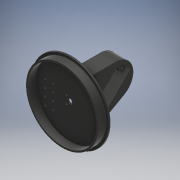
# Autodesk Inventor part: 第一關節
Saved by Autodesk Inventor 2017 (Build 210142000, 142)
## iProperties
Part Number: 第一關節
Material: 熱塑性塑膠樹脂
Document SubType Name: Modeling
Designer: Brian
Density: 1.28 g/cm^3
Appearance: 平滑 - 黑色
Mass: 82.2152 g
Surface Area: 315.278 cm^2
Volume: 64.2306 cm^3
Author: Brian
Autodesk Inventor part; units mm, degrees
ref_plane "YZ Plane" through (0, 0, 0) normal (1, 0, 0) x (0, 1, 0)
ref_plane "XZ Plane" through (0, 0, 0) normal (0, 1, 0) x (-1, 0, 0)
ref_plane "XY Plane" through (0, 0, 0) normal (0, 0, 1) x (1, 0, 0)
sketch "草圖1" plane through (0, 0, 0) normal (0, 1, 0) x (-1, 0, 0)
  circle A0 centre (0, 0) radius 46.75
  circle A1 centre (0, 0) radius 44.75
  dimension "d0" = 93.5
  dimension "d1" = 2
  constraints: 2 centre point, 2 coincident
  measures "d0" diameter of A0
  measures "d1" radial gap between concentric circles of A0 A1
extrude "擠出1" add sketch "草圖1" along normal blind 10
sketch "草圖2" plane through (0, 10, 0) normal (0, 1, 0) x (1, 0, 0)
  circle A0 centre (0, 0) radius 50
  dimension "d4" = 100
  constraints: 1 centre point, 1 coincident
  measures "d4" diameter of A0
extrude "擠出2" add sketch "草圖2" along normal blind 2
sketch "草圖4" plane through (0, 0, 0) normal (1, 0, 0) x (0, 1, 0)
  line L0 (12, -50) -> (12, 50) projected
  line L1 (12, -25.0248) -> (30.0379, -25.0248)
  line L2 (30.0379, -25.0248) -> (30.0379, 11.7448)
  line L3 (30.0379, 11.7448) -> (12, 11.7448)
  line L4 (12, 11.7448) -> (12, -25.0248)
  line L5 (30.0379, -25.0248) -> (72.4644, 17.4017)
  line L6 (72.4644, 17.4017) -> (54.0796, 35.7864)
  line L7 (54.0796, 35.7864) -> (11.6532, -6.64)
  line L8 (11.6532, -6.64) -> (30.0379, -25.0248)
  point P0 (0, 0)
  dimension "d12" = 45
  dimension "d13" = 26
  dimension "d14" = 60
  constraints: 16 end point, 4 parallel, 2 perpendicular, 2 point on line, 1 horizontal
  measures "d12" angle of L2 L7
  measures "d13" distance of L5.end L6.end
  measures "d14" distance of L1.end L5.end
extrude "擠出4" add sketch "草圖4" along normal blind 5
fillet "圓角1" radius 10 1 edges at (2.5, 30.0379, 11.7448)
fillet "圓角2" radius 10 1 edges at (2.5, 30.0379, -25.0248)
sketch "草圖5" plane through (5, 0, 0) normal (1, 0, 0) x (0, 0, -1)
  line L0 (22.0958, 32.9669) -> (-17.4017, 72.4644) projected
  line L1 (-17.4017, 72.4644) -> (-35.7864, 54.0796) projected
  line L2 (-35.7864, 54.0796) -> (-14.6737, 32.9669) projected
  line L3 (20.7821, 30.0379) -> (-17.4017, 68.2217)
  line L4 (-17.4017, 68.2217) -> (-31.5438, 54.0796)
  line L5 (-31.5438, 54.0796) -> (-12.5524, 35.0882)
  line L6 (-31.5438, 54.0796) -> (-17.4017, 68.2217)
  line L7 (-17.4017, 68.2217) -> (20.7821, 30.0379)
  line L8 (20.7821, 30.0379) -> (6.64, 15.8958)
  line L9 (6.64, 15.8958) -> (-31.5438, 54.0796)
  arc A0 (25.0248, 25.8958) -> (22.0958, 32.9669) centre (15.0248, 25.8958) ccw projected
  line L10 (22.0958, 32.9669) -> (-17.4017, 72.4644) projected
  line L11 (-17.4017, 72.4644) -> (-35.7864, 54.0796) projected
  line L12 (-35.7864, 54.0796) -> (-14.6737, 32.9669) projected
  arc A1 (-11.7448, 25.8958) -> (-14.6737, 32.9669) centre (-21.7448, 25.8958) ccw projected
  line L13 (-11.7448, 25.8958) -> (-11.7448, 12) projected
  line L14 (25.0248, 12) -> (-11.7448, 12) projected
  line L15 (25.0248, 12) -> (25.0248, 25.8958) projected
  point P0 (0, 0)
  dimension "d19" = 20
  dimension "d20" = 54
  dimension "d21" = 54
  constraints: 14 end point, 3 equal length, 1 perpendicular, 2 other
  measures "d19" distance of L3.end L4.end
  measures "d20" distance of L3.start L3.end
  measures "d21" distance between parallel lines of L4 L8
extrude "擠出5" add sketch "草圖5" along normal blind 15
sketch "草圖6" plane through (0, 0, 0) normal (-1, 0, 0) x (0, 0, 1)
  circle A0 centre (12.4519, 49.1298) radius 10.5
  line L0 (12.4519, 49.1298) -> (26.594, 63.272)
  line L1 (17.4017, 72.4644) -> (35.7864, 54.0796) projected
  line L2 (-6.64, 15.8958) -> (-20.7821, 30.0379) projected
  point P0 (0, 0)
  dimension "d24" = 37
  dimension "d25" = 21
  constraints: 2 end point, 1 centre point, 1 midpoint, 1 perpendicular
  measures "d24" distance from line of L2 L0.start
  measures "d25" diameter of A0
extrude "擠出6" cut sketch "草圖6" against normal blind 5
sketch "草圖7" plane through (5, 0, 0) normal (1, 0, 0) x (0, 0, -1)
  line L0 (-17.4017, 68.2217) -> (20.7821, 30.0379) projected
  line L1 (15.9031, 34.917) -> (20.7821, 30.0379)
  line L2 (20.7821, 30.0379) -> (15.1253, 24.3811)
  line L3 (15.1253, 24.3811) -> (10.2462, 29.2601)
  line L4 (10.2462, 29.2601) -> (15.9031, 34.917)
  point P0 (0, 0)
  dimension "d28" = 8
  dimension "d29" = 6.9
  constraints: 8 end point, 2 parallel, 1 collinear, 1 perpendicular, 1 point on line
  measures "d28" distance of L3.end L1.start
  measures "d29" distance of L2.end L3.end
extrude "擠出7" add sketch "草圖7" along normal blind 10.8
sketch "草圖8" plane through (5, 0, 0) normal (1, 0, 0) x (0, 0, -1)
  line L0 (-17.2591, 39.7949) -> (6.64, 15.8958) projected
  line L1 (1.7609, 20.7749) -> (6.64, 15.8958)
  line L2 (6.64, 15.8958) -> (12.2968, 21.5527)
  line L3 (12.2968, 21.5527) -> (7.4178, 26.4317)
  line L4 (7.4178, 26.4317) -> (1.7609, 20.7749)
  point P0 (0, 0)
  dimension "d32" = 8
  dimension "d33" = 6.9
  constraints: 8 end point, 2 parallel, 1 collinear, 1 perpendicular, 1 point on line
  measures "d32" distance of L3.end L1.start
  measures "d33" distance of L2.end L3.end
extrude "擠出8" add sketch "草圖8" along normal blind 10.8
sketch "草圖9" plane through (5, 0, 0) normal (1, 0, 0) x (0, 0, -1)
  line L0 (-17.4017, 68.2217) -> (20.7821, 30.0379) projected
  line L1 (-12.5226, 63.3427) -> (-17.4017, 68.2217)
  line L2 (-17.4017, 68.2217) -> (-23.0585, 62.5649)
  line L3 (-23.0585, 62.5649) -> (-18.1795, 57.6858)
  line L4 (-18.1795, 57.6858) -> (-12.5226, 63.3427)
  line L5 (6.64, 15.8958) -> (-31.5438, 54.0796) projected
  line L6 (-26.6648, 49.2005) -> (-31.5438, 54.0796)
  line L7 (-31.5438, 54.0796) -> (-25.8869, 59.7364)
  line L8 (-25.8869, 59.7364) -> (-21.0079, 54.8574)
  line L9 (-21.0079, 54.8574) -> (-26.6648, 49.2005)
  point P0 (0, 0)
  dimension "d36" = 8
  dimension "d37" = 8
  dimension "d38" = 6.9
  constraints: 16 end point, 5 point on line, 4 parallel, 2 perpendicular, 1 collinear
  measures "d36" distance of L3.end L1.start
  measures "d37" distance of L8.end L6.start
  measures "d38" distance of L7.end L8.end
extrude "擠出9" add sketch "草圖9" along normal blind 10.8
fillet "圓角3" radius 2 2 edges at (10.4, 54.8574, 21.0079) (10.4, 57.6858, 18.1795)
fillet "圓角4" radius 2 2 edges at (10.4, 26.4317, -7.4178) (10.4, 29.2601, -10.2462)
sketch "草圖10" plane through (0, 12, -25.0248) normal (0, 0, -1) x (-1, 0, 0)
  line L0 (0, 13.8958) -> (0, 20.9669) projected
  line L1 (0, 13.8958) -> (6, 13.8958)
  line L2 (6, 13.8958) -> (6, 10.8958)
  line L3 (6, 10.8958) -> (0, 10.8958)
  line L4 (0, 10.8958) -> (0, 13.8958)
  line L5 (6, 10.8958) -> (3, 10.8958)
  line L6 (3, 10.8958) -> (3, 6.4247)
  line L7 (3, 6.4247) -> (6, 6.4247)
  line L8 (6, 6.4247) -> (6, 10.8958)
  line L9 (0, 0) -> (0, 13.8958) projected
  point P0 (0, -12)
  dimension "d43" = 3
  dimension "d44" = 3
  dimension "d45" = 3
  constraints: 16 end point, 4 parallel, 2 horizontal, 2 perpendicular
  measures "d43" distance of L1.end L2.end
  measures "d44" distance of L6.end L7.end
  measures "d45" distance between parallel lines of L9 L6
extrude "擠出10" add sketch "草圖10" against normal blind 3
fillet "圓角6" radius 1 3 edges at (0, 25.8958, -23.5248) (0, 24.3958, -22.0248) (0, 22.8958, -23.5248)
fillet "圓角7" radius 1 5 edges at (-3, 22.8958, -23.5248) (-4.5, 18.4247, -22.0248) (-6, 18.4247, -23.5248) (-4.5, 18.4247, -25.0248) (-3, 18.4247, -23.5248)
sketch "草圖11" plane through (15.8, 0, 0) normal (1, 0, 0) x (0, 0, -1)
  line L0 (-19.028, 62.777) -> (-26.0991, 55.7059)
  line L1 (-26.0991, 55.7059) -> (8.2663, 21.3405)
  line L2 (8.2663, 21.3405) -> (15.3374, 28.4116)
  line L3 (15.3374, 28.4116) -> (-19.028, 62.777)
  line L4 (-17.4017, 68.2217) -> (20.7821, 30.0379) projected
  line L5 (-31.5438, 54.0796) -> (-17.4017, 68.2217) projected
  line L6 (12.2968, 21.5527) -> (15.1253, 24.3811) projected
  point P0 (0, 0)
  dimension "d51" = 10
  dimension "d52" = 5
  dimension "d53" = 2.7
  dimension "d54" = 2.7
  constraints: 8 end point, 3 parallel, 1 perpendicular
  measures "d51" distance between parallel lines of L1 L3
  measures "d52" distance between parallel lines of L4 L3
  measures "d53" distance between parallel lines of L5 L0
  measures "d54" distance between parallel lines of L6 L2
hole "孔1" at (15.8, 62.777, 19.028) at (15.8, 55.7059, 26.0991) at (15.8, 21.3405, -8.2663) at (15.8, 28.4116, -15.3374) direction (-1, 0, 0) diameter 3 depth 8 tip angle 118
fillet "圓角8" radius 5 2 edges at (10, 72.4644, 17.4017) (10, 54.0796, 35.7864)
sketch "草圖12" plane through (0, 12, 0) normal (0, 1, 0) x (1, 0, 0)
  line L0 (36.1789, -23.8614) -> (26.1789, -23.8614)
  line L1 (26.1789, -23.8614) -> (26.1789, -13.8614)
  line L2 (26.1789, -13.8614) -> (36.1789, -13.8614)
  line L3 (36.1789, -13.8614) -> (36.1789, -23.8614)
  point P0 (0, 0)
  dimension "d66" = 10
  dimension "d67" = 10
  constraints: 8 end point, 2 parallel, 1 horizontal, 1 perpendicular
  measures "d66" distance of L2.end L0.start
  measures "d67" distance of L0.start L0.end
extrude "擠出11" cut sketch "草圖12" against normal blind 3
move faces "移動1" translate (0, 0.0707, 0.0707) faces at (18.6, 60.6792, 24.9441)
move faces "移動2" translate (0, -0.0707, -0.0707) faces at (18.6, 22.4955, -13.2396)
sketch "草圖13" plane through (0, 0, 0) normal (-1, 0, 0) x (0, 0, 1)
  circle A0 centre (12.4519, 49.1298) radius 10.5 projected
  circle A1 centre (12.4519, 49.1298) radius 22.5
  line L0 (-7.1398, 60.194) -> (-23.7322, 30.8132)
  arc A2 (-22.0958, 32.9669) -> (-24.9746, 26.8958) centre (-15.0248, 25.8958) ccw projected
  line L1 (34.9519, 49.1298) -> (34.9519, 12)
  line L2 (-23.7322, 30.8132) -> (4.1803, 12)
  line L3 (34.9519, 12) -> (4.1803, 12)
  point P0 (0, 0)
  dimension "d74" = 45
  constraints: 8 end point, 3 point on circle, 2 tangent, 1 centre point, 1 coincident
  measures "d74" diameter of A1
extrude "擠出12" add sketch "草圖13" against normal up to surface (5 mm away)
sketch "草圖14" plane through (5, 12, 34.9519) normal (1, 0, 0) x (0, 0, -1)
  arc A0 (58.6841, 18.8132) -> (57.0477, 20.9669) centre (49.9767, 13.8958) ccw projected
  line L0 (42.0917, 48.194) -> (58.6841, 18.8132) projected
  arc A1 (42.0917, 48.194) -> (0, 37.1298) centre (22.5, 37.1298) ccw projected
  line L1 (0, 0) -> (0, 37.1298) projected
  line L2 (23.2071, 0) -> (0, 0) projected
  line L3 (23.2071, 13.8958) -> (23.2071, 0) projected
  arc A2 (23.2071, 13.8958) -> (20.2782, 20.9669) centre (13.2071, 13.8958) ccw projected
  line L4 (2.701, 38.544) -> (20.2782, 20.9669) projected
  arc A3 (2.701, 45.6151) -> (2.701, 38.544) centre (6.2365, 42.0796) ccw projected
  line L5 (14.0147, 56.9288) -> (2.701, 45.6151) projected
  arc A4 (21.0858, 56.9288) -> (14.0147, 56.9288) centre (17.5503, 53.3933) ccw projected
  line L6 (57.0477, 20.9669) -> (21.0858, 56.9288) projected
  point P0 (34.9519, -12)
extrude "擠出13" add sketch "草圖14" along normal up to surface (15 mm away)
fillet "圓角10" radius 5 3 edges at (20, 12, 4.9636) (10, 12, -25.0248) (10, 12, 34.9519)
sketch "草圖15" plane through (0, 12, 0) normal (0, 1, 0) x (1, 0, 0)
  circle A0 centre (0, 0) radius 7
  line L0 (4.9497, -4.9497) -> (-4.9497, -4.9497)
  line L1 (-4.9497, -4.9497) -> (-4.9497, 4.9497)
  line L2 (-4.9497, 4.9497) -> (4.9497, 4.9497)
  line L3 (4.9497, 4.9497) -> (4.9497, -4.9497)
  line L4 (4.9497, -4.9497) -> (-4.9497, 4.9497) construction
  line L5 (-4.9497, -4.9497) -> (4.9497, 4.9497) construction
  dimension "d80" = 14
  constraints: 12 end point, 2 midpoint, 2 parallel, 2 perpendicular, 1 coincident, 1 horizontal, 3 other
hole "孔2" at (-4.9497, 12, -4.9497) at (-4.9497, 12, 4.9497) direction (0, -1, 0) diameter 3.2 depth 8 tip angle 118
sketch "草圖16" plane through (0, 0, 0) normal (-1, 0, 0) x (0, 0, 1)
  line L0 (-34.1064, 30.3841) -> (-11.6862, 30.3841)
  line L1 (-11.6862, 30.3841) -> (-11.6862, 17.5726)
  line L2 (-11.6862, 17.5726) -> (-34.1064, 17.5726)
  line L3 (-34.1064, 17.5726) -> (-34.1064, 30.3841)
  point P0 (0, 0)
  constraints: 8 end point, 2 parallel, 1 horizontal, 1 perpendicular
extrude "擠出14" cut sketch "草圖16" along normal through all
sketch "草圖18" plane through (0, 12, 0) normal (0, 1, 0) x (1, 0, 0)
  circle A0 centre (-32.4933, 20.4975) radius 1.5
  circle A1 centre (-22.4933, 20.4975) radius 1.5
  line L0 (-32.4933, 20.4975) -> (-22.4933, 20.4975)
  point P0 (0, 0)
  dimension "d94" = 3
  dimension "d95" = 3
  dimension "d96" = 10
  constraints: 2 centre point, 2 end point, 1 horizontal
  measures "d94" diameter of A1
  measures "d95" diameter of A0
  measures "d96" distance of L0.start L0.end
extrude "擠出16" cut sketch "草圖18" against normal blind 10
pattern_linear "矩形陣列1" count 4 spacing 10 along (0, 0, 1) of "擠出16"
move faces "移動3" translate (0, 0.1414, -0.1414) faces at (12.2, 36.5901, 14.0543)
move faces "移動4" translate (0, -0.1414, 0.1414) faces at (8.6, 44.1511, -6.6689)
sketch "草圖19" plane through (0, 10, 0) normal (0, -1, 0) x (1, 0, 0)
  circle A0 centre (0, 0) radius 3.25
  dimension "d108" = 6.5
  constraints: 1 centre point, 1 coincident
  measures "d108" diameter of A0
extrude "擠出17" cut sketch "草圖19" against normal blind 2.5
move faces "移動5" translate (-0.9, 0, 0) faces at (15.8, 65.0413, 16.061) (15.8, 52.7017, 28.3159) (15.8, 31.4158, -17.5542) (15.8, 19.0762, -5.2993)
